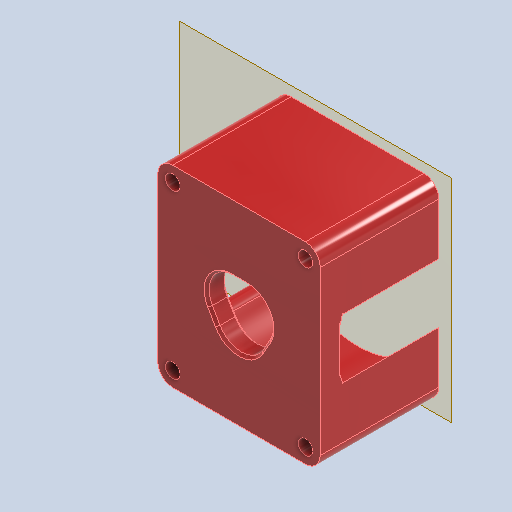
# Autodesk Inventor part: ESP32ParasiteMicroscope_top_v0
Saved by Autodesk Inventor 2022 (Build 260153000, 153)
## iProperties
Created: 2022-02-02
Part Number: ESP32ParasiteMicroscope_top_v0
Material: Generisch
Document SubType Name: Modeling
Designer: diederichbenedict
Density: 1 g/cm^3
Appearance: Rot
Author: diederichbenedict
Autodesk Inventor part; units mm, degrees
ref_plane "YZ Plane" through (0, 0, 0) normal (1, 0, 0) x (0, 1, 0)
ref_plane "XZ Plane" through (0, 0, 0) normal (0, 1, 0) x (-1, 0, 0)
ref_plane "XY Plane" through (0, 0, 0) normal (0, 0, 1) x (1, 0, 0)
ref_plane "Work Plane2" through (-11.007737, 0, -6) normal (0, 0, 1) x (1, 0, 0)
sketch "Sketch5" plane through (-11.007737, 0, -6) normal (0, 0, 1) x (1, 0, 0)
  circle A0 centre (-4.872354, 16.48745) radius 1.45
  circle A1 centre (22, 16.48745) radius 1.45
  circle A2 centre (22, -16.48745) radius 1.45
  circle A3 centre (-4.872354, -16.48745) radius 1.45
  circle A4 centre (8.563823, 0) radius 6
  circle A5 centre (-4.872354, 16.48745) radius 1.45
  circle A6 centre (22, -16.48745) radius 1.45
  circle A7 centre (-4.872354, -16.48745) radius 1.45
  circle A8 centre (22, 16.48745) radius 1.45
  arc A9 (-25, -16.48745) -> (-22, -19.48745) centre (-22, -16.48745) ccw
  line L0 (-22, -19.48745) -> (22, -19.48745)
  arc A10 (22, -19.48745) -> (25, -16.48745) centre (22, -16.48745) ccw
  arc A11 (25, 16.48745) -> (22, 19.48745) centre (22, 16.48745) ccw
  line L1 (22, 19.48745) -> (-22, 19.48745)
  arc A12 (-22, 19.48745) -> (-25, 16.48745) centre (-22, 16.48745) ccw
  line L2 (-25, 16.48745) -> (-25, -16.48745)
  line L3 (-4.872354, -19.48745) -> (22, -19.48745)
  line L4 (25, -16.48745) -> (25, 16.48745)
  line L5 (22, 19.48745) -> (-4.872354, 19.48745)
  line L6 (-7.872354, 16.48745) -> (-7.872354, -16.48745)
  line L7 (-7.872354, -19.48745) -> (25, 19.48745) construction
  line L8 (25, -19.48745) -> (-7.872354, 19.48745) construction
  arc A13 (-4.872354, 19.48745) -> (-7.872354, 16.48745) centre (-4.872354, 16.48745) ccw
  arc A14 (25, 16.48745) -> (22, 19.48745) centre (22, 16.48745) ccw
  arc A15 (22, -19.48745) -> (25, -16.48745) centre (22, -16.48745) ccw
  arc A16 (-7.872354, -16.48745) -> (-4.872354, -19.48745) centre (-4.872354, -16.48745) ccw
  circle A17 centre (8.563823, 0) radius 17.5
  circle A18 centre (-22, 16.48745) radius 1.45
  circle A19 centre (-22, -16.48745) radius 1.45
  line L9 (25, -16.48745) -> (25, 16.48745)
  point P0 (11.007737, 0)
  point P1 (-7.872354, 6.008501)
  point P2 (-7.872354, -6.008501)
  point P3 (25, 6.008501)
  point P4 (25, -6.008501)
  point P5 (-4.872354, -19.48745)
  point P6 (-4.872354, 19.48745)
  dimension "d17" = 3
  dimension "d18" = 35
  constraints: 12 end point, 12 point on circle, 12 point on line, 8 tangent, 5 centre point, 3 equal radius, 2 midpoint, 2 parallel, 1 coincident, 1 horizontal, 1 perpendicular
  measures "d17" radius of A13
  measures "d18" diameter of A17
extrude "Extrusion4" add sketch "Sketch5" along normal blind 20 contours A16 L6 A17 L4 A10 L0 | L1 A11 L4 A17 L6 A13
sketch "Sketch6" plane through (-11.007737, 0, 14) normal (0, 0, 1) x (1, 0, 0)
  line L0 (25, 6.008501) -> (25, 16.48745)
  arc A0 (25, 16.48745) -> (22, 19.48745) centre (22, 16.48745) ccw
  line L1 (22, 19.48745) -> (-4.872354, 19.48745)
  arc A1 (-4.872354, 19.48745) -> (-7.872354, 16.48745) centre (-4.872354, 16.48745) ccw
  line L2 (-7.872354, 16.48745) -> (-7.872354, 6.008501)
  arc A2 (25, 6.008501) -> (-7.872354, 6.008501) centre (8.563823, 0) ccw
  circle A3 centre (-4.872354, 16.48745) radius 1.45
  circle A4 centre (22, 16.48745) radius 1.45
  line L3 (-7.872354, -6.008501) -> (-7.872354, -16.48745)
  arc A5 (-7.872354, -16.48745) -> (-4.872354, -19.48745) centre (-4.872354, -16.48745) ccw
  line L4 (-4.872354, -19.48745) -> (22, -19.48745)
  arc A6 (22, -19.48745) -> (25, -16.48745) centre (22, -16.48745) ccw
  line L5 (25, -16.48745) -> (25, -6.008501)
  arc A7 (25, 6.008501) -> (-7.872354, 6.008501) centre (8.563823, 0) ccw
  circle A8 centre (-4.872354, -16.48745) radius 1.45
  circle A9 centre (22, -16.48745) radius 1.45
  arc A10 (25, 6.008501) -> (-7.872354, 6.008501) centre (8.563823, 0) ccw
  line L6 (25, 6.008501) -> (25, -6.008501)
  arc A11 (-7.872354, -6.008501) -> (25, -6.008501) centre (8.563823, 0) ccw
  line L7 (-7.872354, 6.008501) -> (-7.872354, -6.008501)
  circle A12 centre (8.563823, 0) radius 6 construction
  circle A13 centre (8.563823, 0) radius 5.9 construction
  line L8 (7.004977, 5.9) -> (10.122669, 5.9)
  line L9 (14.452796, -1.6) -> (12.89395, -4.3)
  line L10 (4.233696, -4.3) -> (2.67485, -1.6)
  arc A14 (7.004977, 5.9) -> (2.67485, -1.6) centre (7.004977, 0.9) ccw
  arc A15 (14.452796, -1.6) -> (10.122669, 5.9) centre (10.122669, 0.9) ccw
  arc A16 (4.233696, -4.3) -> (12.89395, -4.3) centre (8.563823, -1.8) ccw
  arc A17 (-7.872354, -6.008501) -> (25, -6.008501) centre (8.563823, 0) ccw
  line L11 (-7.872354, 16.48745) -> (-7.872354, 6.008501)
  line L12 (25, 6.008501) -> (25, 16.48745)
  arc A18 (25, 16.48745) -> (22, 19.48745) centre (22, 16.48745) ccw
  line L13 (22, 19.48745) -> (-4.872354, 19.48745)
  arc A19 (-4.872354, 19.48745) -> (-7.872354, 16.48745) centre (-4.872354, 16.48745) ccw
  line L14 (25, -16.48745) -> (25, -6.008501)
  arc A20 (-7.872354, -6.008501) -> (25, -6.008501) centre (8.563823, 0) ccw
  line L15 (-7.872354, -6.008501) -> (-7.872354, -16.48745)
  arc A21 (-7.872354, -16.48745) -> (-4.872354, -19.48745) centre (-4.872354, -16.48745) ccw
  line L16 (-4.872354, -19.48745) -> (22, -19.48745)
  arc A22 (22, -19.48745) -> (25, -16.48745) centre (22, -16.48745) ccw
  point P0 (11.007737, 0)
  point P1 (-1.655277, 5.9)
  point P2 (18.782923, 5.9)
  point P3 (8.563823, -11.8)
  dimension "d24" = 11.8
  dimension "d28" = 5
  constraints: 10 end point, 7 point on circle, 7 point on line, 7 tangent, 4 centre point, 2 coincident, 2 collinear, 2 equal radius, 1 parallel, 7 other
  measures "d24" diameter of A13
  measures "d28" radius of A14
extrude "Extrusion5" add sketch "Sketch6" along normal blind 4
fillet "Fillet1" radius 2 2 edges at (-18.8801, 6.0085, 4) (-18.8801, -6.0085, 4)
chamfer "Chamfer1" distance 0.5 angle 45 16 edges at (-8.3329, 3.4, 18) (-2.4439, 5.9, 18) (3.4451, 3.4, 18) (2.6656, -2.95, 18) (-2.4439, -6.8, 18) (-7.5535, -2.95, 18) (-8.3329, 3.4, 14) (-2.4439, 5.9, 14) (3.4451, 3.4, 14) (2.6656, -2.95, 14) (-2.4439, -6.8, 14) (-7.5535, -2.95, 14) (0.9194, 17.1738, 14) (0.9194, -17.1738, 14) (-17.6008, 11.2434, 14) (-17.6008, -11.2434, 14)
body "Solid2"
